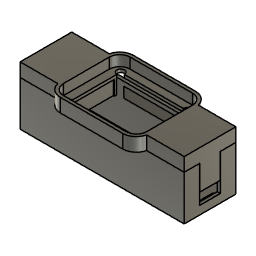
MacSniffer_Case (Autodesk Fusion 360 design; units mm, degrees)
Autodesk Fusion 360 part; units mm, degrees
sketch "Sketch1" plane through (0, 0, 0) normal (0, 0, 1) x (1, 0, 0)
  line L0 (37.9, -10.9) -> (-37.9, -10.9)
  line L1 (-37.9, -10.9) -> (-37.9, 10.9)
  line L2 (-37.9, 10.9) -> (37.9, 10.9)
  line L3 (37.9, 10.9) -> (37.9, -10.9)
  line L4 (37.9, -10.9) -> (-37.9, 10.9) construction
  line L5 (-37.9, -10.9) -> (37.9, 10.9) construction
  line L6 (-37.9, 0) -> (37.9, 0) construction
  circle A0 centre (35.9, 5.7) radius 1
  circle A1 centre (35.9, -5.7) radius 1
  line L7 (39.4, -12.4) -> (-39.4, -12.4)
  line L8 (-39.4, -12.4) -> (-39.4, 12.4)
  line L9 (-39.4, 12.4) -> (39.4, 12.4)
  line L10 (39.4, 12.4) -> (39.4, -12.4)
  line L11 (-37.9, 9) -> (-39.4, 9)
  line L12 (37.9, 5) -> (39.4, 5)
  line L13 (37.9, -5) -> (39.4, -5)
  line L14 (-37.9, -9) -> (-39.4, -9)
  dimension "d1" = 75.8
  dimension "d2" = 21.8
  dimension "d3" = 2
  dimension "d4" = 2
  dimension "d5" = 5.7
  dimension "d15" = 9
  dimension "d16" = 5
  constraint horizontal L0
  constraint perpendicular L0 L1
  constraint parallel L0 L2
  constraint parallel L1 L3
  constraint coincident L4 origin
  constraint coincident L5 origin
  constraint midpoint L1 L6.start
  constraint midpoint L3 L6.end
  constraint symmetric L6 A0 A1
  constraint coincident L1 L11.start
  constraint coincident L8 L11.end
  constraint perpendicular L8 L11
  constraint coincident L3 L12.start
  constraint coincident L10 L12.end
  constraint perpendicular L10 L12
  constraint symmetric L6 L12.start L13.start
  constraint symmetric L6 L12.end L13.end
  constraint symmetric L6 L11.start L14.start
  constraint symmetric L6 L11.end L14.end
  measures "d1" distance of L1.end L2.end
  measures "d2" distance of L0.end L1.end
  measures "d3" diameter of A0
  measures "d4" distance of L3 A0.centre
  measures "d5" distance of L6 A0.centre
  measures "d15" distance of L6 L11
  measures "d16" distance of L6 L12
extrude "Extrude1" add sketch "Sketch1" against normal blind 1.5 contours L0 L1 L3 L7 L8 L10 L13 L14 | L0 L1 L2 L3 | L3 L10 L12 L13 | L1 L8 L11 L14 | L1 L2 L3 L8 L9 L10 L11 L12 | A0 | A1 makes body 1
extrude "Extrude2" add sketch "Sketch1" along normal blind 20 contours L0 L1 L3 L7 L8 L10 L13 L14 | L1 L2 L3 L8 L9 L10 L11 L12 bodies 1
extrude "Extrude3" add sketch "Sketch1" along normal blind 2.5 contours L3 L10 L12 L13 | L1 L8 L11 L14 bodies 1
sketch "Sketch1 (1)" plane through (0, 10.9, 0) normal (0, -1, 0) x (1, 0, 0)
  line L0 (-37.9, 0) -> (37.9, 0)
  line L1 (37.9, 0) -> (37.9, 20)
  line L2 (37.9, 20) -> (-37.9, 20)
  line L3 (-37.9, 20) -> (-37.9, 0)
  line L4 (-12.9, 18) -> (33.9, 18)
  line L5 (33.9, 18) -> (33.9, 13)
  line L6 (33.9, 13) -> (-12.9, 13)
  line L7 (-12.9, 13) -> (-12.9, 18)
  dimension "d21" = 25
  dimension "d22" = 4
  dimension "d23" = 2
  dimension "d24" = 5
  constraint horizontal L4
  constraint vertical L5
  constraint horizontal L6
  constraint vertical L7
  measures "d21" distance of L3 L7
  measures "d22" distance of L1 L5
  measures "d23" distance of L2 L4
  measures "d24" distance of L4.end L5.end
ref_plane "WorkPlane1" through (0, 0, 10) normal (0, -1, 0) x (1, 0, 0)
extrude "Extrude4" add sketch "Sketch1 (1)" along normal blind 7 draft -45 contours L4 L5 L6 L7 bodies 1
mirror "Mirror1" about plane through (0, 0, 10) normal (0, -1, 0) of "Extrude4"
sketch "Sketch2" plane through (0, 0, 20) normal (0, 0, 1) x (-1, 0, 0)
  line L0 (37.9, -9) -> (37.9, -10.9)
  line L1 (37.9, -10.9) -> (-37.9, -10.9)
  line L2 (-37.9, -10.9) -> (-37.9, -5)
  line L3 (-37.9, -5) -> (-39.4, -5)
  line L4 (-39.4, -5) -> (-39.4, -12.4)
  line L5 (-39.4, -12.4) -> (39.4, -12.4)
  line L6 (39.4, -12.4) -> (39.4, -9)
  line L7 (39.4, -9) -> (37.9, -9)
  line L8 (-37.9, 5) -> (-37.9, 10.9)
  line L9 (-37.9, 10.9) -> (37.9, 10.9)
  line L10 (37.9, 10.9) -> (37.9, 9)
  line L11 (37.9, 9) -> (39.4, 9)
  line L12 (39.4, 9) -> (39.4, 12.4)
  line L13 (39.4, 12.4) -> (-39.4, 12.4)
  line L14 (-39.4, 12.4) -> (-39.4, 5)
  line L15 (-39.4, 5) -> (-37.9, 5)
  line L16 (39.4, -9) -> (39.4, 9)
  line L17 (-39.4, -5) -> (-39.4, 5)
  line L18 (-37.9, -5) -> (-37.9, 5)
  line L19 (37.9, -9) -> (37.9, 9)
  line L20 (37.5, -9) -> (37.5, -10.5)
  line L21 (37.5, -10.5) -> (-37.5, -10.5)
  line L22 (-37.5, -10.5) -> (-37.5, -5)
  line L23 (-37.5, -5) -> (-37.5, 5)
  line L24 (-37.5, 5) -> (-37.5, 10.5)
  line L25 (-37.5, 10.5) -> (37.5, 10.5)
  line L26 (37.5, 10.5) -> (37.5, 9)
  line L27 (37.5, -9) -> (37.5, 9)
  line L28 (37.5, 10.5) -> (35.5, 10.5)
  line L29 (35.5, 10.5) -> (35.5, 8.5)
  line L30 (35.5, 8.5) -> (37.5, 8.5)
  line L31 (37.5, 8.5) -> (37.5, 10.5)
  line L32 (37.5, -10.5) -> (35.5, -10.5)
  line L33 (35.5, -10.5) -> (35.5, -8.5)
  line L34 (35.5, -8.5) -> (37.5, -8.5)
  line L35 (37.5, -8.5) -> (37.5, -10.5)
  line L36 (37.9, 9) -> (37.5, 9)
  line L37 (37.9, -9) -> (37.5, -9)
  line L38 (35.5, 8.5) -> (35.5, -8.5)
  dimension "d29" = 0.4
  dimension "d50" = 2
  dimension "d51" = 2
  dimension "d52" = 2
  dimension "d53" = 2
  constraint coincident L6.end L7.start
  constraint coincident L11.end L12.start
  constraint coincident L3.end L4.start
  constraint coincident L14.end L15.start
  constraint coincident L2.end L3.start
  constraint coincident L8.start L15.end
  constraint coincident L0.start L7.end
  constraint coincident L10.end L11.start
  constraint horizontal L28
  constraint vertical L29
  constraint horizontal L30
  constraint vertical L31
  constraint horizontal L32
  constraint vertical L33
  constraint horizontal L34
  constraint vertical L35
  constraint perpendicular L27 L36
  constraint perpendicular L27 L37
  measures "d50" distance of L25.end L28.end
  measures "d51" distance of L25.end L30.end
  measures "d52" distance of L20.end L32.end
  measures "d53" distance of L20.end L34.end
extrude "Extrude5" add sketch "Sketch2" along normal blind 1.5 separate body makes body 2
extrude "Extrude6" add sketch "Sketch2" against normal blind 7 contours L20 L21 L27 L32 L33 L34 L35 | L25 L26 L27 L28 L29 L30 L31 | L27 L30 L34 L38 | L21 L22 L23 L24 L25 L29 L33 L38 bodies 2
extrude "Extrude7" cut 1 faces at (-37.5, 3.5, 15.3333) along direction (1, 0, 0) blind 20 on bodies 2 bodies 2
extrude "Extrude8" cut sketch "Sketch1 (1)" along normal blind 3.7 draft -45 from surface at 0.4 contours L4 L5 L6 L7 bodies 2
mirror "Mirror2" about plane through (0, 0, 10) normal (0, -1, 0) of "Extrude8"
shell "Shell1" thickness 1 removed faces 1 at (2.7, 3.5, 13) on bodies 2
extrude "Extrude9" add sketch "Sketch2" against normal blind 12 contours L3 L15 L17 L18 bodies 2
move_face "OffsetFaces1" offset -0.1 2 faces at (38.9, -5, 16) (38.4, 5, 16) on bodies 2
extrude "Extrude10" add 1 faces at (37.9, 1.6333, 16) along direction (-1, 0, 0) up to surface (0.4 mm away) on bodies 2 bodies 2
extrude "Extrude11" add sketch "Sketch2" against normal blind 1.5 contours L7 L11 L16 L19 bodies 2
move_face "OffsetFaces2" offset -0.1 2 faces at (-38.4, -9, 19.5) (-38.9, 9, 19.5) on bodies 2
extrude "Extrude12" add sketch "Sketch2" against normal up to surface (1.5 mm away) contours L19 L27 L31 L35 L36 L37 | L20 L21 L27 L32 L33 L34 L35 | L25 L26 L27 L28 L29 L30 L31 | L27 L30 L34 L38 bodies 2
sketch "Sketch3" plane through (0, 0, 0) normal (0, 0, 1) x (-1, 0, 0)
  line L0 (-37.9, 10.9) -> (-37.9, -10.9)
  line L1 (-37.9, -10.9) -> (37.9, -10.9)
  line L2 (37.9, -10.9) -> (37.9, 10.9)
  line L3 (37.9, 10.9) -> (-37.9, 10.9)
  line L4 (-35.9, -5) -> (-37.9, -5)
  line L5 (-37.9, -5) -> (-37.9, 5.0147)
  line L6 (-37.9, 5.0147) -> (-35.9, 5.0147)
  line L7 (-35.9, 5.0147) -> (-35.9, -5)
  line L8 (-37.9, -5) -> (-37.9, 5)
  line L9 (-37.9, -5) -> (-39.4, -5)
  dimension "d56" = 2
  constraint horizontal L4
  constraint vertical L5
  constraint horizontal L6
  constraint vertical L7
  constraint collinear L5 L8
  constraint collinear L4 L9
  measures "d56" distance of L4.start L4.end
extrude "Extrude13" add sketch "Sketch3" along normal blind 1 contours L0 L4 L5 L6 L7 L8 bodies 1
sketch "Display" plane through (0, 0, 21.5) normal (0, 0, 1) x (-1, 0, 0)
  line L0 (-39.4, -12.4) -> (39.4, -12.4)
  line L1 (39.4, -12.4) -> (39.4, 12.4)
  line L2 (39.4, 12.4) -> (-39.4, 12.4)
  line L3 (-39.4, 12.4) -> (-39.4, -12.4)
  line L4 (-15, 16) -> (15, 16)
  line L5 (20, 11) -> (20, -11)
  line L6 (15, -16) -> (-15, -16)
  line L7 (-20, -11) -> (-20, 11)
  line L8 (-20, 16) -> (20, -16) construction
  line L9 (20, 16) -> (-20, -16) construction
  line L10 (-16, 12.5) -> (16, 12.5)
  line L11 (16, 12.5) -> (16, -12.5)
  line L12 (16, -12.5) -> (-16, -12.5)
  line L13 (-16, -12.5) -> (-16, 12.5)
  line L14 (-16, 12.5) -> (16, -12.5) construction
  line L15 (16, 12.5) -> (-16, -12.5) construction
  circle A0 centre (16, -12.5) radius 1.85
  circle A1 centre (-16, -12.5) radius 1.85
  circle A2 centre (-16, 12.5) radius 1.85
  circle A3 centre (16, 12.5) radius 1.85
  arc A4 (15, -16) -> (20, -11) centre (15, -11) ccw
  arc A5 (-20, -11) -> (-15, -16) centre (-15, -11) ccw
  arc A6 (-15, 16) -> (-20, 11) centre (-15, 11) ccw
  arc A7 (20, 11) -> (15, 16) centre (15, 11) ccw
  line L16 (15, -17.5) -> (-15, -17.5)
  arc A8 (-21.5, -11) -> (-15, -17.5) centre (-15, -11) ccw
  line L17 (-21.5, -11) -> (-21.5, 11)
  arc A9 (-15, 17.5) -> (-21.5, 11) centre (-15, 11) ccw
  line L18 (-15, 17.5) -> (15, 17.5)
  arc A10 (21.5, 11) -> (15, 17.5) centre (15, 11) ccw
  line L19 (21.5, 11) -> (21.5, -11)
  arc A11 (15, -17.5) -> (21.5, -11) centre (15, -11) ccw
  dimension "d59" = 40
  dimension "d60" = 32
  dimension "d61" = 32
  dimension "d62" = 25
  dimension "d63" = 3.7
  dimension "d65" = 3.7
  dimension "d66" = 3.7
  dimension "d67" = 3.7
  dimension "d68" = 5
  dimension "d69" = 5
  dimension "d70" = 5
  dimension "d71" = 5
  constraint horizontal L4
  constraint perpendicular L4 L5
  constraint parallel L4 L6
  constraint parallel L5 L7
  constraint coincident L8 origin
  constraint coincident L9 origin
  constraint horizontal L10
  constraint perpendicular L10 L11
  constraint parallel L10 L12
  constraint parallel L11 L13
  constraint coincident L14 origin
  constraint coincident L15 origin
  constraint coincident L11.end L12.start
  constraint coincident L12.end L13.start
  constraint coincident L10.start L13.end
  constraint coincident L10.end L11.start
  constraint coincident L8.end L6
  constraint coincident L8.end L5
  constraint tangent L6 A4
  constraint tangent L5 A4
  constraint coincident L9.end L6
  constraint coincident L9.end L7
  constraint tangent L6 A5
  constraint tangent L7 A5
  constraint coincident L8.start L4
  constraint coincident L8.start L7
  constraint tangent L4 A6
  constraint tangent L7 A6
  constraint coincident L9.start L5
  constraint coincident L9.start L4
  constraint tangent L5 A7
  constraint tangent L4 A7
  measures "d59" distance of L8.end L9.end
  measures "d60" distance of L9.start L8.end
  measures "d61" distance of L11.end L12.end
  measures "d62" distance of L10.end L11.end
  measures "d63" diameter of A0
  measures "d65" diameter of A1
  measures "d66" diameter of A2
  measures "d67" diameter of A3
  measures "d68" radius of A4
  measures "d69" radius of A5
  measures "d70" radius of A6
  measures "d71" radius of A7
copy_body "CopyPasteBodies1" bodies 2 makes body 3
move_body "Move1" bodies 3 to x (1, 0, 0) y (0, 1, 0) z (0, 0, 1) at (0, 0, 0)
extrude "Extrude14" add sketch "Display" along normal blind 6 contours L0 L2 L7 A5 A6 A8 L17 A9 | L0 L6 A4 A5 L16 A8 A11 | L2 L4 A6 A7 A9 L18 A10 | L0 L2 L5 A4 A7 A10 L19 A11 bodies 3
extrude "Extrude15" add sketch "Display" against normal up to surface (1.5 mm away) contours L0 L6 A4 A5 L16 A8 A11 | L0 L2 L7 L13 A1 A2 A5 A6 | L0 L6 L12 A0 A1 A4 A5 | L2 L4 A6 A7 A9 L18 A10 | L0 L13 A1 | L0 L12 L13 A1 | L2 L4 L10 A2 A3 A6 A7 | L0 L12 L13 A1 | L0 L12 A0 A1 | L2 L10 L13 A2 | L2 L13 A2 | L0 L11 L12 A0 | L0 L11 L12 A0 | L0 L2 L5 L11 A0 A3 A4 A7 | L2 L10 L13 A2 | L2 L10 A2 A3 | L0 L11 A0 | L2 L10 L11 A3 | L2 L10 L11 A3 | L2 L11 A3 picked at (-17.2211, -12.3157) picked at (-17.2211, 12.3157) picked at (17.2211, -12.3157) picked at (17.2211, 12.3157) bodies 3
extrude "Extrude17" add 2 faces at (27.1333, 3.1667, 21.5) (-33.4333, -3.6667, 21.5) along direction (0, 0, 1) up to surface end surface through (0, 0, 27.5) normal (0, 0, 1) offset 0 on bodies 3 bodies 3
extrude "Extrude18" cut sketch "Display" against normal blind 23 contours L0 L13 A1 | L0 L2 L11 L13 A0 A1 A2 A3 | L2 L13 A2 | L0 L11 A0 | L2 L11 A3 picked at (-14.7789, -12.3157) picked at (-14.7789, 12.3157) picked at (14.7789, -12.3157) picked at (14.7789, 12.3157) bodies 3
extrude "Extrude19" cut sketch "Display" against normal up to surface (1.5 mm away) contours L0 L13 A1 | L0 L12 L13 A1 | L0 L13 A1 | L0 L12 L13 A1 | L2 L10 L13 A2 | L2 L13 A2 | L2 L13 A2 | L0 L11 L12 A0 | L0 L11 L12 A0 | L2 L10 L13 A2 | L0 L11 A0 | L0 L11 A0 | L2 L10 L11 A3 | L2 L10 L11 A3 | L2 L11 A3 | L2 L11 A3 bodies 3
extrude "Extrude20" cut 1 faces at (-32.9333, 3.6667, 27.5) along direction (0, 0, -1) blind 1 on bodies 3 bodies 3
hidden bodies 2
equation "d1 = board_length + 2 * clearance"
equation "d2 = board_width + 2 * clearance"
equation "d5 = ( 11.4 / 2 ) * 1 mm"
equation "board_width = 21 mm"
equation "board_length = 75 mm"
equation "clearance = 0.4 mm"
equation "wall_thickness = 1.5 mm"
equation "d10 = -wall_thickness"
equation "d13 = -wall_thickness"
equation "d29 = clearance"
equation "d30 = wall_thickness"
equation "d63 = hole_size"
equation "hole_size = 3.7 mm"
equation "d65 = hole_size"
equation "d66 = hole_size"
equation "d67 = hole_size"
equation "d68 = display_radius"
equation "d69 = display_radius"
equation "d70 = display_radius"
equation "d71 = display_radius"
equation "display_radius = 5 mm"
equation "d73 = -wall_thickness"
named bodies: "Bottom", "Top", "Top-Display"
